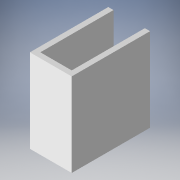
# Autodesk Inventor part: 15102898-16-P-0311
Saved by Autodesk Inventor 2017 (Build 210142000, 142)
## iProperties
Created: 2016-11-06
Part Number: 15102898-16-P-0311
Material: Generic
Document SubType Name: Modeling
Designer: gus
Mass: 17.0562 g
Surface Area: 118.562 cm^2
Volume: 17.0562 cm^3
Density: 1 g/cm^3
Appearance: Default
Author: gus
Autodesk Inventor part; units mm, degrees
ref_plane "YZ Plane" through (0, 0, 0) normal (1, 0, 0) x (0, 1, 0)
ref_plane "XZ Plane" through (0, 0, 0) normal (0, 1, 0) x (-1, 0, 0)
ref_plane "XY Plane" through (0, 0, 0) normal (0, 0, 1) x (1, 0, 0)
sketch "Sketch1" plane through (0, 0, 0) normal (0, 1, 0) x (-1, 0, 0)
  line L0 (0, 0) -> (0, -47.625)
  line L1 (0, -47.625) -> (-3.175, -47.625)
  line L2 (-3.175, -47.625) -> (-3.175, -3.175)
  line L3 (-3.175, -3.175) -> (-22.225, -3.175)
  line L4 (-22.225, -3.175) -> (-22.225, -47.625)
  line L5 (-22.225, -47.625) -> (-25.4, -47.625)
  line L6 (-25.4, -47.625) -> (-25.4, 0)
  line L7 (-25.4, 0) -> (0, 0)
  dimension "d0" = 3.175
  dimension "d1" = 47.625
  dimension "d2" = 3.175
  dimension "d3" = 25.4
  dimension "d4" = 3.175
  constraints: 16 end point, 6 perpendicular, 2 point on line, 1 vertical
  measures "d0" distance of L4.end L5.end
  measures "d1" distance of L5.end L6.end
  measures "d2" distance between parallel lines of L7 L3
  measures "d3" distance of L6.end L0.start
  measures "d4" distance between parallel lines of L0 L2
extrude "Extrusion1" add sketch "Sketch1" along normal blind 50.8
sketch "Sketch2" plane through (25.4, 0, 0) normal (1, 0, 0) x (0, 0, -1)
  line L0 (47.625, 0) -> (47.625, 50.8) projected
  line L1 (47.625, 0) -> (0, 0) projected
  point P0 (38.1, 25.4)
  dimension "d7" = 9.525
  dimension "d8" = 25.4
  measures "d7" distance from line of L0 point (38.1, 25.4)
  measures "d8" distance from line of L1 point (38.1, 25.4)
hole "Hole1" at (25.4, 25.4, -38.1) direction (-1, 0, 0) diameter 6.7469 end through all
chamfer "Chamfer1" distance 19.05 angle 45 2 edges at (1.5875, 50.8, -47.625) (23.8125, 50.8, -47.625)
body "Solid1"
